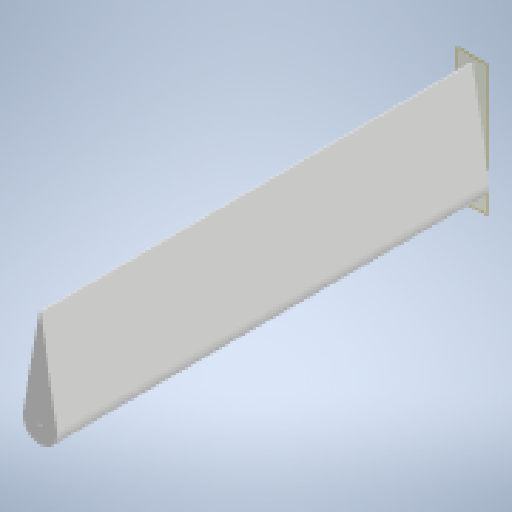
# Autodesk Inventor part: Vtail
Saved by Autodesk Inventor 2026 (Build 300175050, 175E)
## iProperties
Created: 2025-08-11
Part Number: Vtail
Material: Generic
Document SubType Name: Modeling
Designer: Cupri
Mass: 320.314 g
Surface Area: 562.402 cm^2
Volume: 320.314 cm^3
Density: 1 g/cm^3
Appearance: Default
Author: Cupri
Autodesk Inventor part; units mm, degrees
ref_plane "YZ Plane" through (0, 0, 0) normal (1, 0, 0) x (0, 1, 0)
ref_plane "XZ Plane" through (0, 0, 0) normal (0, 1, 0) x (-1, 0, 0)
ref_plane "Work Plane1" through (0, 0, 0) normal (0, 0, 1) x (1, 0, 0)
sketch "Sketch1" plane through (0, 0, 0) normal (0, 0, 1) x (1, 0, 0)
  circle A0 centre (-0.378, 7.3806) radius 0.75 projected
  line L0 (-0.756, 75) -> (0, 75) construction
  arc A1 (-13.4366, 0) -> (12.6806, 0) centre (-0.378, 7.3806) ccw construction
  arc A2 (-12.1028, 9.8588) -> (11.3464, 9.8606) centre (-0.378, 7.3806) ccw
  line L1 (-12.3298, 8.256) -> (-11.557, 13.7119)
  line L2 (11.5739, 8.2546) -> (10.8008, 13.7119)
  line L3 (-12.3298, 8.256) -> (-0.756, 75)
  line L4 (-0.756, 75) -> (0, 75)
  line L5 (0, 75) -> (11.5739, 8.2546)
  spline S0 degree 3 poles (0, 75) (0.0654, 74.6898) (0.2183, 73.9622) (0.6185, 72.0374) (0.8255, 71.0325) (1.5395, 67.5353) (2.0401, 65.0263) (3.7365, 56.3358) (4.8865, 50.1031) (8.482, 29.574) (10.8053, 14.5022) (12.6806, 0) knots -7.652768 -7.652768 -7.652768 -7.652768 -7.375677 -7.375677 -7.074889 -7.074889 -6.315253 -6.315253 -4.432937 -4.432937 -0.050389 -0.050389 -0.050389 -0.050389 projected
  spline S1 degree 3 poles (-13.4366, 0) (-10.3976, 23.501) (-6.0464, 49.5688) (-0.9743, 73.9622) (-0.8214, 74.6898) (-0.756, 75) knots -2.513741 -2.513741 -2.513741 -2.513741 -0.095109 -0.095109 0 0 0 0 projected
  point P0 (0, 0)
  constraints: 10 end point, 4 point on circle, 2 point on line, 1 centre point, 1 collinear
ref_plane "Work Plane2" through (-14.7431, -7.9324, 300) normal (0, 0, -1) x (0, 1, 0)
extrude "Extrusion1" add sketch "Sketch1" along normal up to surface (300 mm away) contours L3 L4 L5 A2
body "Solid1"
